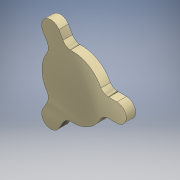
# Autodesk Inventor part: ET1
Saved by Autodesk Inventor 2016 (Build 200138000, 138)
## iProperties
Created: 2016-03-19
Part Number: ET1
Material: Genérico
Document SubType Name: Modeling
Designer: Usuario1
Density: 1 g/cm^3
Appearance: Valor por defecto
Author: Usuario1
Autodesk Inventor part; units mm, degrees
ref_plane "YZ Plane" through (0, 0, 0) normal (1, 0, 0) x (0, 1, 0)
ref_plane "XZ Plane" through (0, 0, 0) normal (0, 1, 0) x (-1, 0, 0)
ref_plane "XY Plane" through (0, 0, 0) normal (0, 0, 1) x (1, 0, 0)
sketch "Boceto1" plane through (0, 0, 0) normal (0, 1, 0) x (-1, 0, 0)
  arc A0 (-2.5488, 0.5326) -> (-2.5488, -0.5326) centre (-2.5488, 0) ccw
  circle A1 centre (-2.5488, 0) radius 0.2
  arc A2 (1.7357, 1.941) -> (0.8131, 2.4736) centre (1.2744, 2.2073) ccw
  circle A3 centre (1.2744, 2.2073) radius 0.2
  line L0 (-2.5488, 0.5326) -> (-2.2825, 0.5326)
  line L1 (-2.5488, -0.5326) -> (-2.2825, -0.5326)
  line L2 (0.8131, 2.4736) -> (0.6799, 2.243)
  line L3 (1.7357, 1.941) -> (1.6025, 1.7103)
  arc A4 (0.8131, -2.4736) -> (1.7357, -1.941) centre (1.2744, -2.2073) ccw
  circle A5 centre (1.2744, -2.2073) radius 0.2
  line L4 (1.7357, -1.941) -> (1.4977, -1.5289)
  arc A6 (1.4642, -1.0203) -> (1.4977, -1.5289) centre (1.9968, -1.2406) ccw
  circle A7 centre (0, 0) radius 0.8
  circle A8 centre (0, 0) radius 1.2
  arc A9 (0.5752, -2.0615) -> (0.1515, -1.7782) centre (0.076, -2.3496) ccw
  line L5 (0.5752, -2.0615) -> (0.8131, -2.4736)
  line L6 (-2.5488, -0.5326) -> (-2.0728, -0.5327)
  arc A10 (-1.6158, -0.7579) -> (-2.0728, -0.5327) centre (-2.0728, -1.109) ccw
  arc A11 (-2.0729, 0.5326) -> (-1.6158, 0.7579) centre (-2.0728, 1.109) ccw
  line L7 (-2.0729, 0.5326) -> (-2.5488, 0.5326)
  line L8 (0.8131, 2.4736) -> (0.5752, 2.0615)
  arc A12 (0.1515, 1.7782) -> (0.5752, 2.0615) centre (0.076, 2.3496) ccw
  arc A13 (1.4977, 1.5289) -> (1.4642, 1.0203) centre (1.9968, 1.2406) ccw
  line L9 (1.4977, 1.5289) -> (1.7357, 1.941)
  arc A14 (-1.6158, -0.7579) -> (0.1515, -1.7782) centre (0, 0) ccw
  arc A15 (0.1515, 1.7782) -> (-1.6158, 0.7579) centre (0, 0) ccw
  arc A16 (1.4642, -1.0203) -> (1.4642, 1.0203) centre (0, 0) ccw
  point P0 (0, 0)
  constraints: 24 point on circle, 20 end point, 17 centre point, 4 point on line
extrude "Extrusión1" add sketch "Boceto1" along normal blind 0.55 contours L0 L7 A11 A15 A12 L8 L2 A2 L3 L9 A13 A16 A6 L4 A4 L5 A9 A14 A10 L6 L1 A0 | A8
sketch "Boceto2" plane through (0, 0.55, 0) normal (0, 1, 0) x (1, 0, 0)
  arc A0 (2.5488, -0.5326) -> (2.5488, 0.5326) centre (2.5488, 0) ccw
  circle A1 centre (2.5488, 0) radius 0.2
  arc A2 (-1.7357, -1.941) -> (-0.8131, -2.4736) centre (-1.2744, -2.2073) ccw
  circle A3 centre (-1.2744, -2.2073) radius 0.2
  line L0 (2.5488, -0.5326) -> (2.2825, -0.5326)
  line L1 (2.5488, 0.5326) -> (2.2825, 0.5326)
  line L2 (-0.8131, -2.4736) -> (-0.6799, -2.243)
  line L3 (-1.7357, -1.941) -> (-1.6025, -1.7103)
  arc A4 (-0.8131, 2.4736) -> (-1.7357, 1.941) centre (-1.2744, 2.2073) ccw
  circle A5 centre (-1.2744, 2.2073) radius 0.2
  line L4 (-1.7357, 1.941) -> (-1.4977, 1.5289)
  arc A6 (-1.4642, 1.0203) -> (-1.4977, 1.5289) centre (-1.9968, 1.2406) ccw
  circle A7 centre (0, 0) radius 0.8
  circle A8 centre (0, 0) radius 1.2
  arc A9 (-0.5752, 2.0615) -> (-0.1515, 1.7782) centre (-0.076, 2.3496) ccw
  line L5 (-0.5752, 2.0615) -> (-0.8131, 2.4736)
  line L6 (2.5488, 0.5326) -> (2.0728, 0.5327)
  arc A10 (1.6158, 0.7579) -> (2.0728, 0.5327) centre (2.0728, 1.109) ccw
  arc A11 (2.0728, -0.5326) -> (1.6158, -0.7579) centre (2.0728, -1.109) ccw
  line L7 (2.0728, -0.5326) -> (2.5488, -0.5326)
  line L8 (-0.8131, -2.4736) -> (-0.5752, -2.0615)
  arc A12 (-0.1515, -1.7782) -> (-0.5752, -2.0615) centre (-0.076, -2.3496) ccw
  arc A13 (-1.4977, -1.5289) -> (-1.4642, -1.0203) centre (-1.9968, -1.2406) ccw
  line L9 (-1.4977, -1.5289) -> (-1.7357, -1.941)
  arc A14 (1.6158, 0.7579) -> (-0.1515, 1.7782) centre (0, 0) ccw
  arc A15 (-0.1515, -1.7782) -> (1.6158, -0.7579) centre (0, 0) ccw
  arc A16 (-1.4642, 1.0203) -> (-1.4642, -1.0203) centre (0, 0) ccw
  constraints: 24 point on circle, 20 end point, 17 centre point, 4 point on line
extrude "Extrusión2" add sketch "Boceto2" along normal blind 0.15 contours A8
sketch "Boceto3" plane through (0, 0, 0) normal (0, 1, 0) x (-1, 0, 0)
  arc A0 (-2.5488, 0.5326) -> (-2.5488, -0.5326) centre (-2.5488, 0) ccw
  circle A1 centre (-2.5488, 0) radius 0.2
  arc A2 (1.7357, 1.941) -> (0.8131, 2.4736) centre (1.2744, 2.2073) ccw
  circle A3 centre (1.2744, 2.2073) radius 0.2
  line L0 (-2.5488, 0.5326) -> (-2.2825, 0.5326)
  line L1 (-2.5488, -0.5326) -> (-2.2825, -0.5326)
  line L2 (0.8131, 2.4736) -> (0.6799, 2.243)
  line L3 (1.7357, 1.941) -> (1.6025, 1.7103)
  arc A4 (0.8131, -2.4736) -> (1.7357, -1.941) centre (1.2744, -2.2073) ccw
  circle A5 centre (1.2744, -2.2073) radius 0.2
  line L4 (1.7357, -1.941) -> (1.4977, -1.5289)
  arc A6 (1.4642, -1.0203) -> (1.4977, -1.5289) centre (1.9968, -1.2406) ccw
  circle A7 centre (0, 0) radius 0.8
  circle A8 centre (0, 0) radius 1.2
  arc A9 (0.5752, -2.0615) -> (0.1515, -1.7782) centre (0.076, -2.3496) ccw
  line L5 (0.5752, -2.0615) -> (0.8131, -2.4736)
  line L6 (-2.5488, -0.5326) -> (-2.0728, -0.5327)
  arc A10 (-1.6158, -0.7579) -> (-2.0728, -0.5327) centre (-2.0728, -1.109) ccw
  arc A11 (-2.0729, 0.5326) -> (-1.6158, 0.7579) centre (-2.0728, 1.109) ccw
  line L7 (-2.0729, 0.5326) -> (-2.5488, 0.5326)
  line L8 (0.8131, 2.4736) -> (0.5752, 2.0615)
  arc A12 (0.1515, 1.7782) -> (0.5752, 2.0615) centre (0.076, 2.3496) ccw
  arc A13 (1.4977, 1.5289) -> (1.4642, 1.0203) centre (1.9968, 1.2406) ccw
  line L9 (1.4977, 1.5289) -> (1.7357, 1.941)
  arc A14 (-1.6158, -0.7579) -> (0.1515, -1.7782) centre (0, 0) ccw
  arc A15 (0.1515, 1.7782) -> (-1.6158, 0.7579) centre (0, 0) ccw
  arc A16 (1.4642, -1.0203) -> (1.4642, 1.0203) centre (0, 0) ccw
  point P0 (0, 0)
  constraints: 24 point on circle, 20 end point, 17 centre point, 4 point on line
extrude "Extrusión3" add sketch "Boceto3" along normal blind 0.2 contours A1 | A3 | A5
sketch "Boceto4" plane through (0, 0, 0) normal (0, -1, 0) x (1, 0, 0)
  arc A0 (1.6158, 0.7579) -> (-0.1515, 1.7782) centre (0, 0) ccw projected
  circle A1 centre (0, 0) radius 0.8 projected
  arc A2 (2.5488, -0.5326) -> (2.5488, 0.5326) centre (2.5488, 0) ccw projected
  line L0 (2.0729, 0.5326) -> (2.5488, 0.5326) projected
  arc A3 (1.6158, 0.7579) -> (2.0729, 0.5326) centre (2.0728, 1.109) ccw projected
  arc A4 (1.6158, 0.7579) -> (-0.1515, 1.7782) centre (0, 0) ccw projected
  arc A5 (-0.5752, 2.0615) -> (-0.1515, 1.7782) centre (-0.076, 2.3496) ccw projected
  line L1 (-0.8131, 2.4736) -> (-0.5752, 2.0615) projected
  arc A6 (-0.8131, 2.4736) -> (-1.7357, 1.941) centre (-1.2744, 2.2073) ccw projected
  line L2 (-1.4977, 1.5289) -> (-1.7357, 1.941) projected
  arc A7 (-1.4642, 1.0203) -> (-1.4977, 1.5289) centre (-1.9968, 1.2406) ccw projected
  arc A8 (-1.4642, 1.0203) -> (-1.4642, -1.0203) centre (0, 0) ccw projected
  arc A9 (-1.4977, -1.5289) -> (-1.4642, -1.0203) centre (-1.9968, -1.2406) ccw projected
  line L3 (-1.7357, -1.941) -> (-1.4977, -1.5289) projected
  arc A10 (-1.7357, -1.941) -> (-0.8131, -2.4736) centre (-1.2744, -2.2073) ccw projected
  line L4 (-0.5752, -2.0615) -> (-0.8131, -2.4736) projected
  arc A11 (-0.1515, -1.7782) -> (-0.5752, -2.0615) centre (-0.076, -2.3496) ccw projected
  arc A12 (-0.1515, -1.7782) -> (1.6158, -0.7579) centre (0, 0) ccw projected
  arc A13 (2.0728, -0.5327) -> (1.6158, -0.7579) centre (2.0728, -1.109) ccw projected
  line L5 (2.5488, -0.5326) -> (2.0728, -0.5327) projected
  line L6 (2.0728, 0.3826) -> (2.5488, 0.3826)
  arc A14 (2.5488, -0.3826) -> (2.5488, 0.3826) centre (2.5488, 0) ccw
  line L7 (2.5488, -0.3826) -> (2.0728, -0.3827)
  arc A15 (2.0728, -0.3827) -> (1.4863, -0.6806) centre (2.0728, -1.109) ccw
  arc A16 (-0.1537, -1.6274) -> (1.4863, -0.6806) centre (0, 0) ccw
  arc A17 (-0.1537, -1.6274) -> (-0.705, -1.9864) centre (-0.076, -2.3496) ccw
  line L8 (-0.705, -1.9864) -> (-0.943, -2.3986)
  arc A18 (-1.6058, -2.016) -> (-0.943, -2.3986) centre (-1.2744, -2.2073) ccw
  line L9 (-1.6058, -2.016) -> (-1.3678, -1.6038)
  arc A19 (-1.3678, -1.6038) -> (-1.3326, -0.9468) centre (-1.9968, -1.2406) ccw
  arc A20 (-1.3326, 0.9468) -> (-1.3326, -0.9468) centre (0, 0) ccw
  arc A21 (-1.3326, 0.9468) -> (-1.3678, 1.6038) centre (-1.9968, 1.2406) ccw
  line L10 (-1.3678, 1.6038) -> (-1.6058, 2.016)
  arc A22 (-0.943, 2.3986) -> (-1.6058, 2.016) centre (-1.2744, 2.2073) ccw
  line L11 (-0.943, 2.3986) -> (-0.705, 1.9864)
  arc A23 (-0.705, 1.9864) -> (-0.1537, 1.6274) centre (-0.076, 2.3496) ccw
  arc A24 (1.4863, 0.6806) -> (-0.1537, 1.6274) centre (0, 0) ccw
  arc A25 (1.4863, 0.6806) -> (2.0728, 0.3826) centre (2.0728, 1.109) ccw
  circle A26 centre (0, 0) radius 0.95
  point P0 (0, 0)
  dimension "d6" = 0.15
  dimension "d7" = 0.15
  constraints: 24 point on circle, 13 centre point, 12 end point, 17 other
  measures "d6" radial gap between concentric circles of A3 A25
  measures "d7" radial gap between concentric circles of A1 A26
extrude "Extrusión4" cut sketch "Boceto4" against normal blind 0.45 contours L6 A14 L7 A15 A16 A17 L8 A18 L9 A19 A20 A21 L10 A22 L11 A23 A24 A25
sketch "Boceto5" plane through (0, 0, 0) normal (0, -1, 0) x (1, 0, 0)
  circle A0 centre (-1.2744, -2.2073) radius 0.2 projected
  circle A1 centre (-1.2744, 2.2073) radius 0.2 projected
  circle A2 centre (2.5488, 0) radius 0.2 projected
  circle A3 centre (-1.2744, -2.2073) radius 0.3
  circle A4 centre (-1.2744, 2.2073) radius 0.3
  circle A5 centre (2.5488, 0) radius 0.3
  point P0 (0, 0)
  dimension "d10" = 0.1
  dimension "d11" = 0.1
  dimension "d12" = 0.1
  constraints: 3 centre point
  measures "d10" radial gap between concentric circles of A0 A3
  measures "d11" radial gap between concentric circles of A1 A4
  measures "d12" radial gap between concentric circles of A2 A5
extrude "Extrusión5" add sketch "Boceto5" against normal blind 0.45
sketch "Boceto6" plane through (0, 0, 0) normal (0, -1, 0) x (1, 0, 0)
  arc A0 (2.5488, -0.5326) -> (2.5488, 0.5326) centre (2.5488, 0) ccw projected
  line L0 (2.0729, 0.5326) -> (2.5488, 0.5326) projected
  arc A1 (1.6158, 0.7579) -> (2.0729, 0.5326) centre (2.0728, 1.109) ccw projected
  arc A2 (1.6158, 0.7579) -> (-0.1515, 1.7782) centre (0, 0) ccw projected
  arc A3 (-0.5752, 2.0615) -> (-0.1515, 1.7782) centre (-0.076, 2.3496) ccw projected
  line L1 (-0.8131, 2.4736) -> (-0.5752, 2.0615) projected
  arc A4 (-0.8131, 2.4736) -> (-1.7357, 1.941) centre (-1.2744, 2.2073) ccw projected
  line L2 (-1.4977, 1.5289) -> (-1.7357, 1.941) projected
  arc A5 (-1.4642, 1.0203) -> (-1.4977, 1.5289) centre (-1.9968, 1.2406) ccw projected
  arc A6 (-1.4642, 1.0203) -> (-1.4642, -1.0203) centre (0, 0) ccw projected
  arc A7 (-1.4977, -1.5289) -> (-1.4642, -1.0203) centre (-1.9968, -1.2406) ccw projected
  line L3 (-1.7357, -1.941) -> (-1.4977, -1.5289) projected
  arc A8 (-1.7357, -1.941) -> (-0.8131, -2.4736) centre (-1.2744, -2.2073) ccw projected
  line L4 (-0.5752, -2.0615) -> (-0.8131, -2.4736) projected
  arc A9 (-0.1515, -1.7782) -> (-0.5752, -2.0615) centre (-0.076, -2.3496) ccw projected
  arc A10 (-0.1515, -1.7782) -> (1.6158, -0.7579) centre (0, 0) ccw projected
  arc A11 (2.0728, -0.5327) -> (1.6158, -0.7579) centre (2.0728, -1.109) ccw projected
  line L5 (2.5488, -0.5326) -> (2.0728, -0.5327) projected
  arc A12 (1.4863, 0.6806) -> (2.0728, 0.3826) centre (2.0728, 1.109) ccw projected
  line L6 (2.0728, 0.3826) -> (2.5488, 0.3826) projected
  arc A13 (2.5488, -0.3826) -> (2.5488, 0.3826) centre (2.5488, 0) ccw projected
  line L7 (2.5488, -0.3826) -> (2.0728, -0.3827) projected
  arc A14 (2.0728, -0.3827) -> (1.4863, -0.6806) centre (2.0728, -1.109) ccw projected
  arc A15 (-0.1537, -1.6274) -> (1.4863, -0.6806) centre (0, 0) ccw projected
  arc A16 (-0.1537, -1.6274) -> (-0.705, -1.9864) centre (-0.076, -2.3496) ccw projected
  line L8 (-0.705, -1.9864) -> (-0.943, -2.3986) projected
  arc A17 (-1.6058, -2.016) -> (-0.943, -2.3986) centre (-1.2744, -2.2073) ccw projected
  line L9 (-1.6058, -2.016) -> (-1.3678, -1.6038) projected
  arc A18 (-1.3678, -1.6038) -> (-1.3326, -0.9468) centre (-1.9968, -1.2406) ccw projected
  arc A19 (-1.3326, 0.9468) -> (-1.3326, -0.9468) centre (0, 0) ccw projected
  arc A20 (-1.3326, 0.9468) -> (-1.3678, 1.6038) centre (-1.9968, 1.2406) ccw projected
  line L10 (-1.3678, 1.6038) -> (-1.6058, 2.016) projected
  arc A21 (-0.943, 2.3986) -> (-1.6058, 2.016) centre (-1.2744, 2.2073) ccw projected
  line L11 (-0.943, 2.3986) -> (-0.705, 1.9864) projected
  arc A22 (-0.705, 1.9864) -> (-0.1537, 1.6274) centre (-0.076, 2.3496) ccw projected
  arc A23 (1.4863, 0.6806) -> (-0.1537, 1.6274) centre (0, 0) ccw projected
  point P0 (0, 0)
extrude "Extrusión6" add sketch "Boceto6" against normal blind 0.15 contours A12 L6 A13 L7 A14 A15 A16 L8 A17 L9 A18 A19 A20 L10 A21 L11 A22 A23
